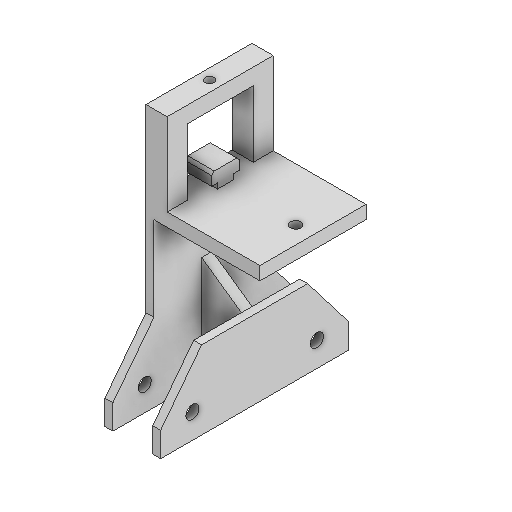
# Autodesk Inventor part: równoważnia
Saved by Autodesk Inventor 2025.1 (Build 291241000, 241)
## iProperties
Created: 2025-04-08
Part Number: równoważnia
Material: Ogólny
Document SubType Name: Modeling
Designer: Maciej
Density: 1 g/cm^3
Appearance: Domyślna
Author: Maciej
Autodesk Inventor part; units mm, degrees
ref_plane "YZ Plane" through (0, 0, 0) normal (1, 0, 0) x (0, 1, 0)
ref_plane "XZ Plane" through (0, 0, 0) normal (0, 1, 0) x (-1, 0, 0)
ref_plane "XY Plane" through (0, 0, 0) normal (0, 0, 1) x (1, 0, 0)
sketch "Szkic1" plane through (0, 0, 0) normal (1, 0, 0) x (0, 1, 0)
  line L0 (81.6216, 12.5) -> (106.6216, 12.5)
  line L1 (106.6216, 12.5) -> (106.6216, -12.5)
  line L2 (106.6216, -12.5) -> (81.6216, -12.5)
  line L3 (81.6216, -12.5) -> (81.6216, 12.5)
  line L4 (81.6216, 12.5) -> (106.6216, -12.5) construction
  line L5 (106.6216, 12.5) -> (81.6216, -12.5) construction
  line L6 (112.7335, 0) -> (112.7335, 20)
  line L7 (112.7335, 20) -> (44.7131, 20)
  line L8 (44.7131, 20) -> (24.5326, 35.4833)
  line L9 (24.5326, 35.4833) -> (15.2555, 35.4833)
  line L10 (15.2555, 35.4833) -> (15.2555, 0)
  line L11 (112.7335, 0) -> (112.7335, -20)
  line L12 (112.7335, -20) -> (44.7131, -20)
  line L13 (44.7131, -20) -> (24.5326, -35.4833)
  line L14 (24.5326, -35.4833) -> (15.2555, -35.4833)
  line L15 (15.2555, -35.4833) -> (15.2555, 0)
  point P0 (0, 0)
  point P1 (94.1216, 0)
  point P2 (24.5326, 19.6832)
  point P3 (24.5326, -19.6832)
  dimension "d0" = 25
  dimension "d1" = 25
  dimension "d2" = 82.089
  dimension "d3" = 20
  constraints: 32 end point, 4 parallel, 3 perpendicular, 2 midpoint, 1 horizontal
  measures "d0" distance of L1.end L2.end
  measures "d1" distance of L0.end L1.end
  measures "d2" distance from line of point (24.533, 19.683) L1
  measures "d3" distance of L6.start L6.end
extrude "Wyciągnięcie proste1" add sketch "Szkic1" along normal blind 3
sketch "Szkic2" plane through (3, 0, 0) normal (1, 0, 0) x (0, 0, -1)
  line L0 (-12.5, 106.6216) -> (12.5, 106.6216) projected
  line L1 (-35.4833, 24.5326) -> (-35.4833, 15.2555) projected
  line L2 (35.4833, 15.2555) -> (35.4833, 24.5326) projected
  point P0 (0, 0)
  point P1 (-23.4833, 24.5326)
  point P2 (23.4833, 24.5326)
  dimension "d6" = 82.089
  dimension "d7" = 82.089
  dimension "d8" = 12
  dimension "d9" = 12
  measures "d6" distance from line of L0 point (-23.483, 24.533)
  measures "d7" distance from line of L0 point (23.483, 24.533)
  measures "d8" distance from line of L1 point (-23.483, 24.533)
  measures "d9" distance from line of L2 point (23.483, 24.533)
hole "Otwór1" at (3, 24.5326, 23.4833) at (3, 24.5326, -23.4833) direction (-1, 0, 0) diameter 5 depth 3 tip angle 118 clearance for "Śruba ze łbem płaskim obrobiona" size "M4" standard "ANSI Profil metryczny M"
sketch "Szkic3" plane through (3, 0, 0) normal (1, 0, 0) x (0, 0, -1)
  line L0 (-12.5, 106.6216) -> (12.5, 106.6216) projected
  line L1 (-12.5, 106.6216) -> (-20, 106.6216)
  line L2 (-20, 112.7335) -> (-20, 44.7131) projected
  line L3 (-12.5, 81.6216) -> (-12.5, 106.6216) projected
  line L4 (-20, 81.6216) -> (-12.5, 81.6216)
  line L5 (-12.5, 81.6216) -> (-12.5, 106.6216)
  line L6 (12.5, 106.6216) -> (12.5, 81.6216) projected
  line L7 (12.5, 106.6216) -> (12.5, 81.6216)
  line L8 (12.5, 81.6216) -> (20, 81.6216)
  line L9 (20, 81.6216) -> (20, 106.6216)
  line L10 (20, 106.6216) -> (12.5, 106.6216)
  line L11 (20, 44.7131) -> (20, 112.7335) projected
  point P0 (0, 0)
  point P1 (-20, 81.6216)
  dimension "d36" = 0
  constraints: 14 end point, 3 perpendicular, 2 horizontal, 2 point on line, 1 collinear, 1 vertical
  measures "d36" distance between parallel lines of L11 L9
extrude "Wyciągnięcie proste2" add sketch "Szkic3" along normal blind 5
sketch "Szkic5" plane through (3, 0, 0) normal (1, 0, 0) x (0, 0, -1)
  line L0 (-35.4833, 15.2555) -> (35.4833, 15.2555) projected
  line L1 (0, 15.2555) -> (-2, 15.2555)
  line L2 (-2, 15.2555) -> (-2, 55.2555)
  line L3 (-2, 55.2555) -> (2, 55.2555)
  line L4 (2, 55.2555) -> (2, 15.2555)
  line L5 (0, 15.2555) -> (2, 15.2555)
  point P0 (0, 0)
  dimension "d26" = 2
  dimension "d27" = 40
  dimension "d28" = 4
  constraints: 10 end point, 3 perpendicular, 2 point on line, 1 collinear, 1 midpoint
  measures "d26" distance of L1.start L1.end
  measures "d27" distance of L1.end L2.end
  measures "d28" distance of L2.end L3.end
extrude "Wyciągnięcie proste3" add sketch "Szkic5" along normal blind 15
sketch "Szkic6" plane through (18, 0, 0) normal (1, 0, 0) x (0, 0, -1)
  line L0 (-35.4833, 15.2555) -> (35.4833, 15.2555) projected
  line L1 (35.4833, 15.2555) -> (35.4833, 24.5326) projected
  line L2 (-35.4833, 15.2555) -> (35.4833, 15.2555)
  line L3 (35.4833, 15.2555) -> (35.4833, 24.5326)
  line L4 (35.4833, 24.5326) -> (20, 44.7131) projected
  line L5 (35.4833, 24.5326) -> (20, 44.7131)
  line L6 (-20, 44.7131) -> (-35.4833, 24.5326) projected
  line L7 (20, 44.7131) -> (-20, 44.7131)
  line L8 (-35.4833, 24.5326) -> (-35.4833, 15.2555) projected
  line L9 (-20, 44.7131) -> (-35.4833, 24.5326)
  line L10 (-35.4833, 24.5326) -> (-35.4833, 15.2555)
  circle A0 centre (-23.4833, 24.5326) radius 2.5 projected
  circle A1 centre (23.4833, 24.5326) radius 2.5 projected
  point P0 (0, 0)
  constraints: 12 end point, 3 collinear, 2 coincident, 1 horizontal, 1 parallel
extrude "Wyciągnięcie proste4" add sketch "Szkic6" along normal blind 3
chamfer "Faza1" distance 10.542 distance2 15 1 edges at (18, 55.2555, 0) measured on face at (18, 54.7555, 0)
sketch "Szkic7" plane through (3, 0, 0) normal (1, 0, 0) x (0, 0, -1)
  line L0 (-20, 81.6216) -> (-12.5, 81.6216) projected
  line L1 (20, 44.7131) -> (20, 112.7335) projected
  line L2 (-20, 81.6216) -> (20, 81.6216)
  line L3 (20, 81.6216) -> (20, 76.6216)
  line L4 (20, 76.6216) -> (-20, 76.6216)
  line L5 (-20, 76.6216) -> (-20, 81.6216)
  point P0 (0, 0)
  dimension "d37" = 5
  constraints: 8 end point, 2 parallel, 1 horizontal, 1 perpendicular, 1 point on line
  measures "d37" distance of L2.end L3.end
extrude "Wyciągnięcie proste5" add sketch "Szkic7" along normal blind 40
sketch "Szkic8" plane through (0, 81.6216, 12.5) normal (0, 1, 0) x (1, 0, 0)
  point P0 (0, 12.5)
  point P1 (36.4571, 12.5)
hole "Otwór3" at (36.4571, 81.6216, 0) direction (0, -1, 0) diameter 4 depth 5 tip angle 118 clearance for "Śruba ze łbem płaskim obrobiona" size "M4" standard "ANSI Profil metryczny M"
sketch "Szkic9" plane through (3, 0, 0) normal (1, 0, 0) x (0, 0, -1)
  line L0 (20, 112.7335) -> (-20, 112.7335) projected
  line L1 (20, 106.6216) -> (12.5, 106.6216) projected
  line L2 (-20, 112.7335) -> (20, 112.7335)
  line L3 (20, 112.7335) -> (20, 106.6216)
  line L4 (20, 106.6216) -> (-20, 106.6216)
  line L5 (-20, 106.6216) -> (-20, 112.7335)
  point P0 (0, 0)
  constraints: 8 end point, 2 parallel, 1 horizontal, 1 perpendicular
extrude "Wyciągnięcie proste6" add sketch "Szkic9" along normal up to surface (5 mm away)
sketch "Szkic10" plane through (0, 0, 0) normal (-1, 0, 0) x (0, 0, 1)
  line L0 (-3.025, 81.6216) -> (-3.025, 83.6216)
  line L1 (-3.025, 83.6216) -> (-5.25, 83.6216)
  line L2 (-5.25, 83.6216) -> (-5.25, 87.1216)
  line L3 (0, 88.1216) -> (-4.25, 88.1216)
  line L4 (-4.25, 88.1216) -> (-5.25, 87.1216)
  line L5 (0, 88.1216) -> (4.25, 88.1216)
  line L6 (4.25, 88.1216) -> (5.25, 87.1216)
  line L7 (5.25, 83.6216) -> (5.25, 87.1216)
  line L8 (3.025, 83.6216) -> (5.25, 83.6216)
  line L9 (3.025, 81.6216) -> (3.025, 83.6216)
  line L10 (-12.5, 81.6216) -> (12.5, 81.6216) projected
  point P0 (0, 0)
  point P1 (0, 81.6216)
  point P2 (0, 81.6216)
  point P3 (-3.025, 82.6216)
  dimension "d49" = 2
  dimension "d50" = 2.225
  dimension "d51" = 3.5
  dimension "d52" = 4.25
  dimension "d53" = 0
  dimension "d54" = 3.025
  constraints: 20 end point, 3 midpoint, 2 perpendicular, 1 vertical
  measures "d49" distance of L0.start L0.end
  measures "d50" distance of L0.end L2.start
  measures "d51" distance of L2.start L4.end
  measures "d52" distance of L3.start L3.end
  measures "d53" vertical distance of point (0, 81.622) L0.start
  measures "d54" horizontal distance of point (0, 81.622) point (-3.025, 82.622)
extrude "Wyciągnięcie proste7" add sketch "Szkic10" against normal blind 10
sketch "Szkic11" plane through (0, 112.7335, 20) normal (0, 1, 0) x (1, 0, 0)
  point P0 (0, 20)
  point P1 (4, 20)
hole "Otwór4" at (4, 112.7335, 0) direction (0, -1, 0) diameter 3.4 depth 6.1119 tip angle 118 clearance for "Śruba ze łbem płaskim obrobiona" size "M3" standard "ANSI Profil metryczny M"
equation "\"d7\" = d6"
equation "\"d9\" = d8"
